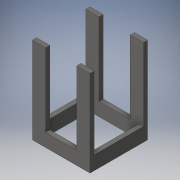
# Autodesk Inventor part: WindShield
Saved by Autodesk Inventor 2016 SP1 (Build 200210100, 210)
## iProperties
Created: 2015-12-18
Part Number: WindShield
Material: Wood (Birch)
Document SubType Name: Modeling
Designer: steele
Density: 0.55 g/cm^3
Appearance: Birch - Natural Polished
Author: steele
Autodesk Inventor part; units mm, degrees
ref_plane "YZ Plane" through (0, 0, 0) normal (1, 0, 0) x (0, 1, 0)
ref_plane "XZ Plane" through (0, 0, 0) normal (0, 1, 0) x (-1, 0, 0)
ref_plane "XY Plane" through (0, 0, 0) normal (0, 0, 1) x (1, 0, 0)
sketch "Sketch1" plane through (0, 0, 0) normal (0, 1, 0) x (-1, 0, 0)
  line L0 (-304.8, 304.8) -> (-304.8, -304.8) construction
  line L1 (-304.8, -304.8) -> (304.8, -304.8) construction
  line L2 (304.8, -304.8) -> (304.8, 304.8) construction
  line L3 (304.8, 304.8) -> (-304.8, 304.8) construction
  line L4 (-304.8, 304.8) -> (304.8, -304.8) construction
  line L5 (-304.8, -304.8) -> (304.8, 304.8) construction
  line L6 (-304.8, 304.8) -> (-165.1, 304.8)
  line L7 (-165.1, 304.8) -> (-165.1, 260.35)
  line L8 (-165.1, 260.35) -> (-304.8, 260.35)
  line L9 (-304.8, 260.35) -> (-304.8, 304.8)
  line L10 (304.8, 304.8) -> (165.1, 304.8)
  line L11 (165.1, 304.8) -> (165.1, 260.35)
  line L12 (165.1, 260.35) -> (304.8, 260.35)
  line L13 (304.8, 260.35) -> (304.8, 304.8)
  line L14 (304.8, -304.8) -> (165.1, -304.8)
  line L15 (165.1, -304.8) -> (165.1, -260.35)
  line L16 (165.1, -260.35) -> (304.8, -260.35)
  line L17 (304.8, -260.35) -> (304.8, -304.8)
  line L18 (-304.8, -304.8) -> (-165.1, -304.8)
  line L19 (-165.1, -304.8) -> (-165.1, -260.35)
  line L20 (-165.1, -260.35) -> (-304.8, -260.35)
  line L21 (-304.8, -260.35) -> (-304.8, -304.8)
  point P0 (0, 0)
  dimension "d0" = 609.6
  dimension "d1" = 609.6
  dimension "d2" = 44.45
  dimension "d3" = 139.7
  constraints: 44 end point, 10 parallel, 5 equal length, 5 perpendicular, 4 horizontal, 2 midpoint, 1 point on line, 1 vertical
  measures "d0" distance of L0.start L0.end
  measures "d1" distance of L2.end L0.start
  measures "d2" distance of L6.end L7.end
  measures "d3" distance of L7.end L8.end
extrude "Extrusion1" add sketch "Sketch1" along normal blind 914.4
sketch "Sketch2" plane through (-165.1, 0, 304.8) normal (1, 0, 0) x (0, 0, -1)
  line L0 (44.45, 0) -> (44.45, 914.4) projected
  line L1 (0, 0) -> (44.45, 0)
  line L2 (44.45, 0) -> (44.45, 139.7)
  line L3 (44.45, 139.7) -> (0, 139.7)
  line L4 (0, 139.7) -> (0, 0)
  line L5 (565.15, 0) -> (565.15, 914.4) projected
  line L6 (609.6, 0) -> (609.6, 914.4) projected
  line L7 (565.15, 0) -> (609.6, 0)
  line L8 (609.6, 0) -> (609.6, 139.7)
  line L9 (609.6, 139.7) -> (565.15, 139.7)
  line L10 (565.15, 139.7) -> (565.15, 0)
  point P0 (304.8, 0)
  dimension "d6" = 139.7
  constraints: 16 end point, 4 parallel, 2 horizontal, 2 perpendicular, 2 point on line, 1 collinear
  measures "d6" distance of L3.end L1.start
extrude "Extrusion2" add sketch "Sketch2" along normal up to next
sketch "Sketch3" plane through (304.8, 0, 260.35) normal (0, 0, -1) x (-1, 0, 0)
  line L0 (0, 0) -> (44.45, 0)
  line L1 (44.45, 0) -> (44.45, 146.2209)
  line L2 (44.45, 146.2209) -> (0, 146.2209)
  line L3 (0, 146.2209) -> (0, 0)
  line L4 (609.6, 0) -> (0, 0) projected
  line L5 (609.6, 0) -> (565.15, 0)
  line L6 (565.15, 0) -> (565.15, 146.2209)
  line L7 (565.15, 146.2209) -> (609.6, 146.2209)
  line L8 (609.6, 146.2209) -> (609.6, 0)
  point P0 (304.8, 0)
  dimension "d9" = 44.45
  constraints: 16 end point, 4 parallel, 2 collinear, 2 horizontal, 2 perpendicular
  measures "d9" distance of L1.end L2.end
extrude "Extrusion3" add sketch "Sketch3" along normal up to next
body "Solid1"
